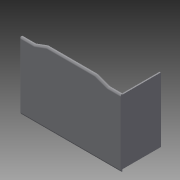
# Autodesk Inventor part: Simple3DPrintBackplate01
Saved by Autodesk Inventor 2015 (Build 190159000, 159)
## iProperties
Created: 2015-09-24
Part Number: Simple3DPrintBackplate01
Material: Generic
Document SubType Name: Modeling
Designer: -
Density: 1 g/cm^3
Appearance: Default
Author: -
Autodesk Inventor part; units mm, degrees
ref_plane "YZ Plane" through (0, 0, 0) normal (1, 0, 0) x (0, 1, 0)
ref_plane "XZ Plane" through (0, 0, 0) normal (0, 1, 0) x (-1, 0, 0)
ref_plane "XY Plane" through (0, 0, 0) normal (0, 0, 1) x (1, 0, 0)
sketch "Sketch1" plane through (0, 0, 0) normal (0, 0, 1) x (1, 0, 0)
  line L0 (56.9468, 33.3564) -> (56.9468, -34.1209) projected
  line L1 (56.9468, -34.1209) -> (-56.9311, -34.1209) projected
  line L2 (-56.9311, -34.1209) -> (-56.9311, 33.3564) projected
  line L3 (-56.9311, 33.3564) -> (-43.6062, 33.3564) projected
  arc A0 (-43.6062, 33.3564) -> (-42.9221, 33.477) centre (-43.6062, 35.3564) ccw projected
  line L4 (-42.9221, 33.477) -> (-30.9163, 37.8468) projected
  arc A1 (-29.5482, 38.088) -> (-30.9163, 37.8468) centre (-29.5482, 34.088) ccw projected
  line L5 (-29.5482, 38.088) -> (19.3938, 38.088) projected
  arc A2 (20.7619, 37.8468) -> (19.3938, 38.088) centre (19.3938, 34.088) ccw projected
  line L6 (20.7619, 37.8468) -> (32.7677, 33.477) projected
  arc A3 (32.7677, 33.477) -> (33.4518, 33.3564) centre (33.4518, 35.3564) ccw projected
  line L7 (33.4518, 33.3564) -> (56.9468, 33.3564) projected
  arc A4 (55.8878, -36.062) -> (58.8878, -33.062) centre (55.8878, -33.062) ccw projected
  line L8 (58.8878, -33.062) -> (58.8878, 31.3564) projected
  arc A5 (58.8878, 31.3564) -> (55.8878, 34.3564) centre (55.8878, 31.3564) ccw projected
  line L9 (55.8878, 34.3564) -> (33.4518, 34.3564) projected
  arc A6 (33.1098, 34.4167) -> (33.4518, 34.3564) centre (33.4518, 35.3564) ccw projected
  line L10 (33.1098, 34.4167) -> (21.1039, 38.7865) projected
  arc A7 (21.1039, 38.7865) -> (19.3938, 39.088) centre (19.3938, 34.088) ccw projected
  line L11 (19.3938, 39.088) -> (-29.5482, 39.088) projected
  arc A8 (-29.5482, 39.088) -> (-31.2583, 38.7865) centre (-29.5482, 34.088) ccw projected
  line L12 (-31.2583, 38.7865) -> (-43.2642, 34.4167) projected
  arc A9 (-43.6062, 34.3564) -> (-43.2642, 34.4167) centre (-43.6062, 35.3564) ccw projected
  line L13 (-43.6062, 34.3564) -> (-56.8722, 34.3564) projected
  arc A10 (-56.8722, 34.3564) -> (-58.8722, 32.3564) centre (-56.8722, 32.3564) ccw projected
  line L14 (-58.8722, 32.3564) -> (-58.8722, -34.062) projected
  arc A11 (-58.8722, -34.062) -> (-56.8722, -36.062) centre (-56.8722, -34.062) ccw projected
  line L15 (-56.8722, -36.062) -> (55.8878, -36.062) projected
  line L16 (-55.9311, 32.3564) -> (-55.9311, -33.1209) projected
  line L17 (-43.6062, 32.3564) -> (-55.9311, 32.3564) projected
  arc A12 (-43.6062, 32.3564) -> (-42.5801, 32.5373) centre (-43.6062, 35.3564) ccw projected
  line L18 (-30.5743, 36.9071) -> (-42.5801, 32.5373) projected
  arc A13 (-29.5482, 37.088) -> (-30.5743, 36.9071) centre (-29.5482, 34.088) ccw projected
  line L19 (19.3938, 37.088) -> (-29.5482, 37.088) projected
  arc A14 (20.4199, 36.9071) -> (19.3938, 37.088) centre (19.3938, 34.088) ccw projected
  line L20 (32.4257, 32.5373) -> (20.4199, 36.9071) projected
  arc A15 (32.4257, 32.5373) -> (33.4518, 32.3564) centre (33.4518, 35.3564) ccw projected
  line L21 (55.9468, 32.3564) -> (33.4518, 32.3564) projected
  line L22 (55.9468, -33.1209) -> (55.9468, 32.3564) projected
  line L23 (-55.9311, -33.1209) -> (55.9468, -33.1209) projected
  line L24 (56.9468, -34.1209) -> (-56.9311, -34.1209) projected
  line L25 (56.9468, 33.3564) -> (56.9468, -34.1209) projected
  line L26 (33.4518, 33.3564) -> (56.9468, 33.3564) projected
  arc A16 (32.7677, 33.477) -> (33.4518, 33.3564) centre (33.4518, 35.3564) ccw projected
  line L27 (20.7619, 37.8468) -> (32.7677, 33.477) projected
  arc A17 (20.7619, 37.8468) -> (19.3938, 38.088) centre (19.3938, 34.088) ccw projected
  line L28 (-29.5482, 38.088) -> (19.3938, 38.088) projected
  arc A18 (-29.5482, 38.088) -> (-30.9163, 37.8468) centre (-29.5482, 34.088) ccw projected
  line L29 (-42.9221, 33.477) -> (-30.9163, 37.8468) projected
  arc A19 (-43.6062, 33.3564) -> (-42.9221, 33.477) centre (-43.6062, 35.3564) ccw projected
  line L30 (-56.9311, 33.3564) -> (-43.6062, 33.3564) projected
  line L31 (-56.9311, -34.1209) -> (-56.9311, 33.3564) projected
  point P0 (0, 0)
extrude "Extrusion1" add sketch "Sketch1" along normal blind 2 contours L0 L1 L2 L3 A0 L4 A1 L5 A2 L6 A3 L7 | L15 A11 L14 A10 L13 A9 L12 A8 L11 A7 L10 A6 L9 A5 L8 A4 | L17 A12 L18 A13 L19 A14 L20 A15 L21 L22 L23 L16
sketch "Sketch3" plane through (0, 0, 0) normal (0, 0, -1) x (-1, 0, 0)
  line L0 (54.9311, 33.3564) -> (43.6062, 33.3564) projected
  line L1 (43.6062, 32.3564) -> (53.9311, 32.3564) projected
  line L2 (30.5743, 36.9071) -> (42.5801, 32.5373) projected
  line L3 (42.9221, 33.477) -> (30.9163, 37.8468) projected
  arc A0 (42.5801, 32.5373) -> (43.6062, 32.3564) centre (43.6062, 35.3564) ccw projected
  arc A1 (42.9221, 33.477) -> (43.6062, 33.3564) centre (43.6062, 35.3564) ccw projected
  arc A2 (55.9311, 30.3564) -> (53.9311, 32.3564) centre (53.9311, 30.3564) ccw projected
  arc A3 (56.9311, 31.3564) -> (54.9311, 33.3564) centre (54.9311, 31.3564) ccw projected
  line L4 (56.9311, -32.1209) -> (56.9311, 31.3564) projected
  line L5 (55.9311, 30.3564) -> (55.9311, -31.1209) projected
  arc A4 (53.9311, -33.1209) -> (55.9311, -31.1209) centre (53.9311, -31.1209) ccw projected
  arc A5 (-54.9468, 33.3564) -> (-56.9468, 31.3564) centre (-54.9468, 31.3564) ccw projected
  line L6 (-33.4518, 33.3564) -> (-54.9468, 33.3564) projected
  arc A6 (-33.4518, 33.3564) -> (-32.7677, 33.477) centre (-33.4518, 35.3564) ccw projected
  line L7 (-20.7619, 37.8468) -> (-32.7677, 33.477) projected
  arc A7 (-19.3938, 38.088) -> (-20.7619, 37.8468) centre (-19.3938, 34.088) ccw projected
  line L8 (29.5482, 38.088) -> (-19.3938, 38.088) projected
  arc A8 (30.9163, 37.8468) -> (29.5482, 38.088) centre (29.5482, 34.088) ccw projected
  line L9 (42.9221, 33.477) -> (30.9163, 37.8468) projected
  arc A9 (42.9221, 33.477) -> (43.6062, 33.3564) centre (43.6062, 35.3564) ccw projected
  line L10 (54.9311, 33.3564) -> (43.6062, 33.3564) projected
  arc A10 (56.9311, 31.3564) -> (54.9311, 33.3564) centre (54.9311, 31.3564) ccw projected
  line L11 (56.9311, -32.1209) -> (56.9311, 31.3564) projected
  arc A11 (54.9311, -34.1209) -> (56.9311, -32.1209) centre (54.9311, -32.1209) ccw projected
  line L12 (-54.9468, -34.1209) -> (54.9311, -34.1209) projected
  arc A12 (-56.9468, -32.1209) -> (-54.9468, -34.1209) centre (-54.9468, -32.1209) ccw projected
  line L13 (-56.9468, 31.3564) -> (-56.9468, -32.1209) projected
  line L14 (43.6062, 32.3564) -> (53.9311, 32.3564) projected
  arc A13 (42.5801, 32.5373) -> (43.6062, 32.3564) centre (43.6062, 35.3564) ccw projected
  line L15 (30.5743, 36.9071) -> (42.5801, 32.5373) projected
  arc A14 (30.5743, 36.9071) -> (29.5482, 37.088) centre (29.5482, 34.088) ccw projected
  line L16 (-19.3938, 37.088) -> (29.5482, 37.088) projected
  arc A15 (-19.3938, 37.088) -> (-20.4199, 36.9071) centre (-19.3938, 34.088) ccw projected
  line L17 (-32.4257, 32.5373) -> (-20.4199, 36.9071) projected
  arc A16 (-33.4518, 32.3564) -> (-32.4257, 32.5373) centre (-33.4518, 35.3564) ccw projected
  line L18 (-53.9468, 32.3564) -> (-33.4518, 32.3564) projected
  arc A17 (-53.9468, 32.3564) -> (-55.9468, 30.3564) centre (-53.9468, 30.3564) ccw projected
  line L19 (-55.9468, -31.1209) -> (-55.9468, 30.3564) projected
  arc A18 (-55.9468, -31.1209) -> (-53.9468, -33.1209) centre (-53.9468, -31.1209) ccw projected
  line L20 (53.9311, -33.1209) -> (-53.9468, -33.1209) projected
  arc A19 (53.9311, -33.1209) -> (55.9311, -31.1209) centre (53.9311, -31.1209) ccw projected
  line L21 (55.9311, 30.3564) -> (55.9311, -31.1209) projected
  arc A20 (55.9311, 30.3564) -> (53.9311, 32.3564) centre (53.9311, 30.3564) ccw projected
  point P0 (0, 0)
extrude "Extrusion2" add sketch "Sketch3" along normal blind 1 contours A3 L4 A11 L12 A12 L13 A5 L6 A6 L7 A7 L8 A8 L3 A1 L0 | L1 A2 L5 A4 L20 A18 L19 A17 L18 A16 L17 A15 L16 A14 L2 A0
chamfer "Chamfer1" distance 1.5 distance2 1 16 edges at (-50.2392, 34.3564, 2) (-58.2864, 33.7706, 2) (-58.8722, -0.8528, 2) (-58.2864, -35.4762, 2) (-0.4922, -36.062, 2) (58.0091, -35.1833, 2) (58.8878, -0.8528, 2) (58.0091, 33.4777, 2) (44.6698, 34.3564, 2) (33.2781, 34.3716, 2) (27.1068, 36.6016, 2) (20.2621, 39.0121, 2) (-5.0772, 39.088, 2) (-30.4165, 39.0121, 2) (-37.2612, 36.6016, 2) (-43.4325, 34.3716, 2) measured on face at (33.1913, 33.8792, 2) measured on face at (44.6698, 33.8564, 2) measured on face at (20.1752, 38.5197, 2) measured on face at (-5.0772, 38.588, 2) measured on face at (-30.3296, 38.5197, 2) measured on face at (-58.3722, -0.8528, 2) measured on face at (57.6556, -34.8297, 2) measured on face at (26.9358, 36.1318, 2) measured on face at (-57.9329, -35.1226, 2) measured on face at (-50.2392, 33.8564, 2) measured on face at (-57.9329, 33.4171, 2) measured on face at (-0.4922, -35.562, 2) measured on face at (57.6556, 33.1242, 2) measured on face at (58.3878, -0.8528, 2) measured on face at (-37.0902, 36.1318, 2) measured on face at (-43.3457, 33.8792, 2)
fillet "Fillet1" radius 2 16 edges at (-43.1721, 32.8944, 2) (-36.7482, 35.1921, 2) (-30.156, 37.5349, 2) (-5.0772, 37.588, 2) (20.0016, 37.5349, 2) (26.5938, 35.1921, 2) (33.0177, 32.8944, 2) (44.6698, 32.8564, 2) (56.9485, 32.4171, 2) (57.3878, -0.8528, 2) (56.9485, -34.1226, 2) (-0.4922, -34.562, 2) (-57.2258, -34.4155, 2) (-57.3722, -0.8528, 2) (-57.2258, 32.71, 2) (-50.2392, 32.8564, 2)
fillet "Fillet2" radius 1 16 edges at (-58.2864, 33.7706, 1) (-58.8722, -0.8528, 1) (-58.2864, -35.4762, 1) (-0.4922, -36.062, 1) (58.0091, -35.1833, 1) (58.8878, -0.8528, 1) (58.0091, 33.4777, 1) (44.6698, 34.3564, 1) (33.2781, 34.3716, 1) (27.1068, 36.6016, 1) (20.2621, 39.0121, 1) (-5.0772, 39.088, 1) (-30.4165, 39.0121, 1) (-37.2612, 36.6016, 1) (-43.4325, 34.3716, 1) (-50.2392, 34.3564, 1)
sketch "Sketch4" plane through (0, 0, 2) normal (0, 0, 1) x (1, 0, 0)
  line L0 (45.7278, -31.062) -> (45.7278, 26.088) projected
  line L1 (88.5778, 61.0907) -> (47.0278, 61.0907)
  line L2 (47.0278, 61.0907) -> (47.0278, -62.6292)
  line L3 (47.0278, -62.6292) -> (88.5778, -62.6292)
  line L4 (88.5778, -62.6292) -> (88.5778, 61.0907)
  point P0 (0, 0)
  dimension "d14" = 1.3
  constraints: 8 end point, 2 parallel, 1 horizontal, 1 perpendicular
  measures "d14" distance between parallel lines of L2 L0
extrude "Extrusion3" cut sketch "Sketch4" against normal blind 10
sketch "Sketch5" plane through (0, 0, -1) normal (0, 0, -1) x (-1, 0, 0)
  line L0 (-47.0278, -34.1209) -> (54.9311, -34.1209) projected
  arc A0 (54.9311, -34.1209) -> (56.9311, -32.1209) centre (54.9311, -32.1209) ccw projected
  line L1 (56.9311, -32.1209) -> (56.9311, 31.3564) projected
  arc A1 (56.9311, 31.3564) -> (54.9311, 33.3564) centre (54.9311, 31.3564) ccw projected
  line L2 (54.9311, 33.3564) -> (43.6062, 33.3564) projected
  arc A2 (42.9221, 33.477) -> (43.6062, 33.3564) centre (43.6062, 35.3564) ccw projected
  line L3 (42.9221, 33.477) -> (30.9163, 37.8468) projected
  arc A3 (30.9163, 37.8468) -> (29.5482, 38.088) centre (29.5482, 34.088) ccw projected
  line L4 (29.5482, 38.088) -> (-19.3938, 38.088) projected
  arc A4 (-19.3938, 38.088) -> (-20.7619, 37.8468) centre (-19.3938, 34.088) ccw projected
  line L5 (-20.7619, 37.8468) -> (-32.7677, 33.477) projected
  arc A5 (-33.4518, 33.3564) -> (-32.7677, 33.477) centre (-33.4518, 35.3564) ccw projected
  line L6 (-33.4518, 33.3564) -> (-47.0278, 33.3564) projected
  line L7 (-47.0278, -34.1209) -> (54.9311, -34.1209) projected
  line L8 (-47.0278, 33.3564) -> (-47.0278, -34.1209) projected
  line L9 (-47.0278, 33.3564) -> (-33.4518, 33.3564) projected
  line L10 (-47.0278, -34.1209) -> (-45.7278, -34.1209)
  line L11 (-45.7278, -34.1209) -> (-45.7278, 33.3564)
  line L12 (-45.7278, 33.3564) -> (-47.0278, 33.3564)
  line L13 (-47.0278, 33.3564) -> (-47.0278, -34.1209)
  point P0 (0, 0)
  point P1 (-45.7278, -34.1209)
  dimension "d15" = 1.3
  constraints: 8 end point, 2 parallel, 1 horizontal, 1 perpendicular, 1 point on line
  measures "d15" distance of L12.end L11.end
extrude "Extrusion4" add sketch "Sketch5" along normal blind 39.08 contours L8 L6 L11 L0
body "Solid1"
